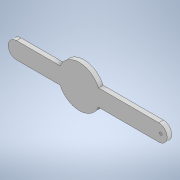
# Autodesk Inventor part: lamina
Saved by Autodesk Inventor 2022 (Build 260153000, 153)
## iProperties
Created: 2022-11-15
Part Number: lamina
Material: Genérico
Document SubType Name: Modeling
Designer: Usuario
Density: 1 g/cm^3
Appearance: Valor por defecto
Author: Usuario
Autodesk Inventor part; units mm, degrees
ref_plane "YZ Plane" through (0, 0, 0) normal (1, 0, 0) x (0, 1, 0)
ref_plane "XZ Plane" through (0, 0, 0) normal (0, 1, 0) x (-1, 0, 0)
ref_plane "XY Plane" through (0, 0, 0) normal (0, 0, 1) x (1, 0, 0)
sketch "Boceto1" plane through (0, 0, 0) normal (0, 0, 1) x (1, 0, 0)
  line L0 (0, 0) -> (-20, 0)
  line L1 (-20, 0) -> (0, 0)
  line L2 (-20, 0) -> (0, 0)
  line L3 (-65, -10) -> (65, -10)
  line L4 (65, -10) -> (65, 10)
  line L5 (65, 10) -> (-65, 10)
  line L6 (-65, 10) -> (-65, -10)
  circle A0 centre (-10, 0) radius 25
  point P0 (-20, -35)
  point P1 (12.9129, 10)
  point P2 (-32.9129, 10)
  point P3 (-32.9129, -10)
  point P4 (12.9129, -10)
  dimension "d4" = 20
  dimension "d6" = 130
  dimension "d7" = 20
  dimension "d8" = 50
  constraints: 14 end point, 4 horizontal, 2 parallel, 1 centre point, 1 midpoint, 1 perpendicular
  measures "d4" distance of L0.start L0.end
  measures "d6" distance of L5.end L4.end
  measures "d7" distance of L4.end L3.end
  measures "d8" diameter of A0
extrude "Extrusión1" add sketch "Boceto1" along normal blind 5.5
sketch "Boceto2" plane through (0, 0, 5.5) normal (0, 0, 1) x (1, 0, 0)
  line L0 (65, -10) -> (65, 10) projected
  line L1 (65, 0) -> (90, 0)
  line L2 (65, 0) -> (85, 0)
  line L3 (85, 0) -> (90, 0)
  circle A0 centre (87.5, 0) radius 1.5
  line L4 (65, 0) -> (95, 0)
  line L5 (95, 0) -> (95, -10)
  line L6 (12.9129, -10) -> (65, -10) projected
  line L7 (95, -10) -> (65, -10)
  line L8 (65, -10) -> (65, 10)
  line L9 (95, 10) -> (65, 10)
  line L10 (95, 0) -> (95, 10)
  arc A1 (95, -2.0554) -> (95, 0) centre (85.9536, -1.0277) ccw
  arc A2 (95, 0) -> (95, 2.0554) centre (85.9536, 1.0277) ccw
  arc A3 (85, -10) -> (85, 10) centre (85, 0) ccw
  point P0 (0, 0)
  point P1 (87.5, -10)
  point P2 (87.5, 10)
  point P3 (95, 2.0554)
  point P4 (87.5, 10)
  point P5 (95, -2.0554)
  dimension "d11" = 25
  dimension "d12" = 20
  dimension "d13" = 3
  dimension "d14" = 30
  constraints: 18 end point, 8 point on line, 6 point on circle, 5 perpendicular, 4 centre point, 3 tangent, 2 midpoint, 2 symmetric about line, 1 collinear, 1 horizontal, 1 other
  measures "d11" distance of L1.start L1.end
  measures "d12" distance of L1.start L2.end
  measures "d13" diameter of A0
  measures "d14" distance of L1.start L4.end
extrude "Extrusión2" add sketch "Boceto2" against normal blind 5.5 contours L0 L1 A0 L4 A3 L7 | L0 L9 A3 L4 L1 A0
sketch "Boceto4" plane through (0, 0, 5.5) normal (0, 0, 1) x (1, 0, 0)
  line L0 (-65, 10) -> (-65, -10) projected
  line L1 (-65, 0) -> (-95, 0)
  line L2 (-95, 0) -> (-95, 10)
  line L3 (-95, 10) -> (-65, 10)
  line L4 (-65, -10) -> (-95, -10)
  line L5 (-95, -10) -> (-95, 0)
  line L6 (-65, 0) -> (-85, 0)
  arc A0 (-85, 10) -> (-85, -10) centre (-85, 0) ccw
  point P0 (0, 0)
  dimension "d17" = 30
  dimension "d18" = 20
  constraints: 12 end point, 3 perpendicular, 3 point on line, 3 tangent, 2 horizontal, 2 point on circle, 1 centre point, 1 midpoint
  measures "d17" distance of L1.start L1.end
  measures "d18" distance of L1.start L6.end
extrude "Extrusión3" add sketch "Boceto4" against normal blind 5.5 contours L0 L1 A0 L3 | L0 L4 A0 L1
